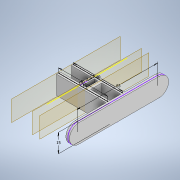
# Autodesk Inventor part: LegMiddle
Saved by Autodesk Inventor 2020.3 (Build 243373000, 373)
## iProperties
Created: 2021-02-16
Part Number: LegMiddle
Material: Generic
Document SubType Name: Modeling
Designer: sanyi
Density: 1 g/cm^3
Appearance: Default
Author: sanyi
Autodesk Inventor part; units mm, degrees
ref_plane "XZ Plane" through (0, 0, 0) normal (0, 1, 0) x (-1, 0, 0)
sketch "Sketch1" plane through (0, 0, 0) normal (1, 0, 0) x (0, 1, 0)
  line L0 (15, 0) -> (15, 32.5)
  line L1 (15, 6) -> (0, 6)
  line L2 (0, 32.5) -> (0, 0)
  line L3 (15, 0) -> (15, 32.5)
  line L4 (15, 6) -> (0, 6)
  line L5 (0, 32.5) -> (0, 0)
  arc A0 (15, 32.5) -> (0, 32.5) centre (7.5, 32.5) ccw
  line L6 (15, 0) -> (0, 0)
  line L7 (15, 0) -> (15, -32.5)
  line L8 (15, -6) -> (0, -6)
  line L9 (0, -32.5) -> (0, 0)
  line L10 (15, -6) -> (0, -6)
  line L11 (15, 0) -> (15, -32.5)
  line L12 (0, -32.5) -> (0, 0)
  arc A1 (0, -32.5) -> (15, -32.5) centre (7.5, -32.5) ccw
  dimension "d25" = 65
  dimension "d26" = 15
  constraints: 26 end point, 8 point on line, 5 symmetric about line, 4 point on circle, 2 centre point, 2 tangent, 1 horizontal, 1 other
  measures "d25" distance of A1.centre A0.centre
  measures "d26" distance of L1.start L1.end
ref_plane "Work Plane1" through (0, 0, 6) normal (0, 0, 1) x (1, 0, 0)
ref_plane "Work Plane2" through (0, 15, -6) normal (0, 0, -1) x (-1, 0, 0)
extrude "Extrusion1" add sketch "Sketch1" along normal mid plane 3
sketch "Sketch2" plane through (0, 0, 6) normal (0, 0, 1) x (1, 0, 0)
  line L0 (-1.5, 15) -> (-41.5, 15)
  line L1 (-41.5, 15) -> (-41.5, 0)
  line L2 (-41.5, 0) -> (-1.5, 0)
  line L3 (-21.5, 15) -> (-21.5, 0)
  line L4 (-18.5, 15) -> (-18.5, 0)
  line L5 (-24.5, 15) -> (-24.5, 0)
  line L6 (-1.5, 15) -> (-1.5, 0)
  line L7 (-1.5, 0) -> (0, 0)
  dimension "d30" = 40
  dimension "d31" = 3
  dimension "d32" = 3
  constraints: 16 end point, 9 perpendicular, 4 point on line, 2 midpoint, 1 horizontal
  measures "d30" distance of L0.start L0.end
  measures "d31" distance between parallel lines of L3 L5
  measures "d32" distance between parallel lines of L3 L4
sketch "Sketch3" plane through (0, 15, -6) normal (0, 0, -1) x (-1, 0, 0)
  line L0 (1.5, -15) -> (1.5, 0) projected
  line L1 (41.5, 0) -> (41.5, -15)
  line L2 (41.5, -15) -> (1.5, -15)
  line L3 (1.5, 0) -> (41.5, 0)
  line L4 (21.5, 0) -> (21.5, -15)
  line L5 (24.5, 0) -> (24.5, -15)
  line L6 (18.5, 0) -> (18.5, -15)
  line L7 (1.5, 0) -> (1.5, -15)
  point P0 (0, -15)
  dimension "d35" = 40
  constraints: 14 end point, 4 point on line, 2 equal length, 2 midpoint, 1 horizontal, 1 perpendicular
  measures "d35" distance of L0.end L1.start
ref_plane "Work Plane5" through (-18.5, 0, 0) normal (1, 0, 0) x (0, 1, 0)
ref_plane "Work Plane6" through (-24.5, 15, 6) normal (1, 0, 0) x (0, 1, 0)
ref_plane "Work Plane7" through (-41.5, 15, 6) normal (1, 0, 0) x (0, 1, 0)
sketch "Sketch5" plane through (-18.5, 0, 0) normal (1, 0, 0) x (0, 1, 0)
  line L0 (15, -32.5) -> (15, 32.5) projected
  line L1 (0, 0) -> (15, 0)
  line L2 (15, 0) -> (15, 6)
  line L3 (15, 6) -> (0, 6)
  line L4 (0, 6) -> (0, 0)
  line L5 (0, 0) -> (15, 0)
  line L6 (15, 0) -> (15, -6)
  line L7 (15, -6) -> (0, -6)
  line L8 (0, -6) -> (0, 0)
  dimension "d42" = 6
  dimension "d43" = 6
  constraints: 16 end point, 4 parallel, 2 horizontal, 2 perpendicular, 2 point on line
  measures "d42" distance of L2.end L1.end
  measures "d43" distance of L5.end L6.end
sketch "Sketch6" plane through (-24.5, 15, 6) normal (1, 0, 0) x (0, 1, 0)
  line L0 (-15, -6) -> (0, -6)
  line L1 (0, -6) -> (0, 0)
  line L2 (0, 0) -> (-15, 0)
  line L3 (-15, 0) -> (-15, -6)
  line L4 (0, -38.5) -> (0, 26.5) projected
  line L5 (-15, -6) -> (0, -6)
  line L6 (0, -6) -> (0, -12)
  line L7 (0, -12) -> (-15, -12)
  line L8 (-15, -12) -> (-15, -6)
  dimension "d44" = 6
  constraints: 16 end point, 4 parallel, 2 horizontal, 2 perpendicular, 1 point on line
  measures "d44" distance of L5.end L6.end
extrude "Extrusion2" add sketch "Sketch2" along normal mid plane 3
extrude "Extrusion3" add sketch "Sketch3" along normal mid plane 3
extrude "Extrusion4" add sketch "Sketch6" along normal mid plane 3
extrude "Extrusion5" add sketch "Sketch5" along normal mid plane 3
body "Solid1"
